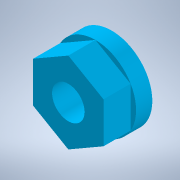
# Autodesk Inventor part: 頭ねじ
Saved by Autodesk Inventor 2020 (Build 240168000, 168)
## iProperties
Created: 2020-03-29
Part Number: 頭ねじ
Material: アルミニウム
Document SubType Name: Modeling
Designer: happy
Density: 2.7 g/cm^3
Appearance: スカイ ブルー 標準
Mass: 2.79358 g
Surface Area: 8.14049 cm^2
Volume: 1.03466 cm^3
Author: happy
Autodesk Inventor part; units mm, degrees
ref_plane "YZ Plane" through (0, 0, 0) normal (1, 0, 0) x (0, 1, 0)
ref_plane "XZ Plane" through (0, 0, 0) normal (0, 1, 0) x (-1, 0, 0)
ref_plane "XY Plane" through (0, 0, 0) normal (0, 0, 1) x (1, 0, 0)
sketch "スケッチ1" plane through (0, 0, 0) normal (0, 0, 1) x (1, 0, 0)
  circle A0 centre (0, 0) radius 7.5
  dimension "d0" = 15
  constraints: 1 centre point, 1 coincident
  measures "d0" diameter of A0
extrude "押し出し1" add sketch "スケッチ1" along normal blind 3
sketch "スケッチ2" plane through (0, 0, 3) normal (0, 0, 1) x (1, 0, 0)
  line L0 (0, 7.5) -> (6.4952, 3.75)
  line L1 (6.4952, 3.75) -> (6.4952, -3.75)
  line L2 (6.4952, -3.75) -> (0, -7.5)
  line L3 (0, -7.5) -> (-6.4952, -3.75)
  line L4 (-6.4952, -3.75) -> (-6.4952, 3.75)
  line L5 (-6.4952, 3.75) -> (0, 7.5)
  point P0 (0, 0)
  point P1 (0, 0)
  dimension "d8" = 7.5
  constraints: 12 end point, 1 coincident, 13 other
  measures "d8" distance of L3.end L4.end
extrude "押し出し2" add sketch "スケッチ2" along normal blind 5
sketch "スケッチ3" plane through (0, 0, 8) normal (0, 0, 1) x (1, 0, 0)
  circle A0 centre (0, 0) radius 3
  dimension "d5" = 6
  constraints: 1 centre point, 1 coincident
  measures "d5" diameter of A0
extrude "押し出し3" cut sketch "スケッチ3" against normal blind 30
